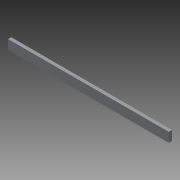
# Autodesk Inventor part: nd-3
Saved by Autodesk Inventor 2015 (Build 190159000, 159)
## iProperties
Created: 2014-07-02
Part Number: nd-3
Material: Generic
Document SubType Name: Modeling
Designer: peter
Density: 1 g/cm^3
Appearance: Default
Author: peter
Autodesk Inventor part; units mm, degrees
ref_plane "YZ Plane" through (0, 0, 0) normal (1, 0, 0) x (0, 1, 0)
ref_plane "XZ Plane" through (0, 0, 0) normal (0, 1, 0) x (-1, 0, 0)
ref_plane "XY Plane" through (0, 0, 0) normal (0, 0, 1) x (1, 0, 0)
sketch "Sketch1" plane through (0, 0, 0) normal (0, 0, 1) x (1, 0, 0)
  line L0 (965.2429, 57.1929) -> (0.0429, 57.1929)
  line L1 (965.2429, 57.1929) -> (0.0429, 57.1929)
  line L2 (0.0429, 57.1929) -> (0.0429, 0.0429)
  line L3 (0.0429, 0.0429) -> (965.2429, 0.0429)
  line L4 (965.2429, 0.0429) -> (965.2429, 57.1929)
  point P0 (0, 0)
  constraints: 10 end point
extrude "Extrusion1" add sketch "Sketch1" along normal blind 19.05
body "Solid1"
